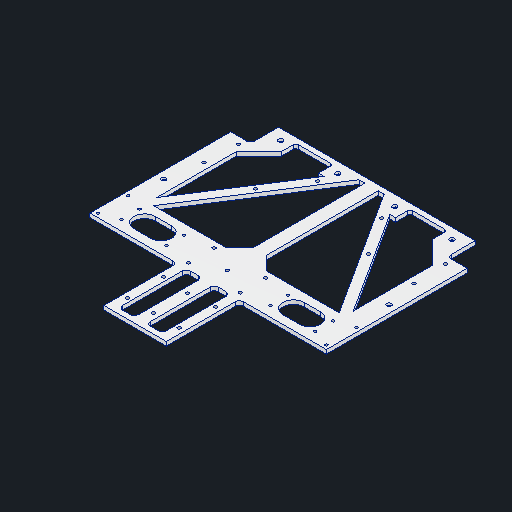
# Autodesk Inventor part: base
Saved by Autodesk Inventor 2023 (Build 270158000, 158)
## iProperties
Created: 2024-04-10
Part Number: base
Material: Aluminum 6061
Document SubType Name: Modeling
Designer: szymo
Density: 2.7 g/cm^3
Appearance: Aluminum - Flat
Mass: 95.625 g
Surface Area: 308.097 cm^2
Volume: 35.4167 cm^3
Author: szymo
Autodesk Inventor part; units mm, degrees
ref_plane "YZ Plane" through (0, 0, 0) normal (1, 0, 0) x (0, 1, 0)
ref_plane "XZ Plane" through (0, 0, 0) normal (0, 1, 0) x (-1, 0, 0)
ref_plane "XY Plane" through (0, 0, 0) normal (0, 0, 1) x (1, 0, 0)
sketch "Sketch2" plane through (0, 0, 0) normal (0, 1, 0) x (-1, 0, 0)
  line L0 (-89, 99) -> (89, 99)
  line L1 (89, 99) -> (89, -99)
  line L2 (89, -99) -> (-89, -99)
  line L3 (-89, -99) -> (-89, 99)
  line L4 (-89, 99) -> (89, -99) construction
  line L5 (89, 99) -> (-89, -99) construction
  line L6 (-89, 99) -> (89, 99)
  line L7 (89, 99) -> (89, -85)
  line L8 (89, -85) -> (-89, -85)
  line L9 (-89, -85) -> (-89, 99)
  line L10 (-4.5, 99) -> (-89, 99)
  line L11 (-89, 99) -> (-89, 42)
  line L12 (-89, 42) -> (-4.5, 42)
  line L13 (-4.5, 42) -> (-4.5, 99)
  line L14 (4.5, 99) -> (89, 99)
  line L15 (89, 99) -> (89, 42)
  line L16 (89, 42) -> (4.5, 42)
  line L17 (4.5, 42) -> (4.5, 99)
  line L18 (22.5, 77.5) -> (22.5, 66.5) projected
  line L19 (16.5, 66.5) -> (16.5, 77.5) projected
  line L20 (-22.5, 66.5) -> (-22.5, 77.5) projected
  line L21 (-16.5, 77.5) -> (-16.5, 66.5) projected
  line L22 (-23.5, 99) -> (-16.5, 99)
  line L23 (-16.5, 99) -> (-16.5, 42)
  line L24 (-16.5, 42) -> (-23.5, 42)
  line L25 (-23.5, 42) -> (-23.5, 99)
  line L26 (16.5, 99) -> (23.5, 99)
  line L27 (23.5, 99) -> (23.5, 42)
  line L28 (23.5, 42) -> (16.5, 42)
  line L29 (16.5, 42) -> (16.5, 99)
  line L30 (-89, 99) -> (89, 99)
  line L31 (89, 99) -> (89, 97)
  line L32 (89, 97) -> (-89, 97)
  line L33 (-89, 97) -> (-89, 99)
  line L34 (89, -85) -> (74, -85)
  line L35 (74, -85) -> (74, -64)
  line L36 (74, -64) -> (89, -64)
  line L37 (89, -64) -> (89, -85)
  line L38 (-89, -85) -> (-74, -85)
  line L39 (-74, -85) -> (-74, -64)
  line L40 (-74, -64) -> (-89, -64)
  line L41 (-89, -64) -> (-89, -85)
  line L42 (16.5, 97) -> (-16.5, 97)
  line L43 (-16.5, 97) -> (-16.5, 93)
  line L44 (-16.5, 93) -> (16.5, 93)
  line L45 (16.5, 93) -> (16.5, 97)
  line L46 (-84.4, -75) -> (-84.4, -71.5) projected
  line L47 (-84.4, -71.5) -> (-87, -71.5) projected
  line L48 (-87, -71.5) -> (-87, -75) projected
  line L49 (-87, -75) -> (-84.4, -75) projected
  line L50 (-79.6, -75) -> (-77, -75) projected
  line L51 (-77, -75) -> (-77, -71.5) projected
  line L52 (-77, -71.5) -> (-79.6, -71.5) projected
  line L53 (-79.6, -71.5) -> (-79.6, -75) projected
  line L54 (-75, -78) -> (-89, -78) projected
  line L55 (-89, -78) -> (-89, -63) projected
  line L56 (-89, -63) -> (-75, -63) projected
  line L57 (-75, -63) -> (-75, -78) projected
  circle A0 centre (-80.45, -67.25) radius 1.25 projected
  point P0 (0, 0)
  point P1 (4.5, 99)
  point P2 (-4.5, 99)
  point P3 (-89, 42)
  point P4 (89, 42)
  point P5 (4.5, 97)
  point P6 (-4.5, 97)
  point P7 (-16.5, 97)
  point P8 (-23.5, 97)
  point P9 (23.5, 97)
  point P10 (16.5, 98)
  point P11 (-4.5, 93)
  point P12 (4.5, 93)
  point P13 (16.5, 93)
  dimension "d8" = 178
  dimension "d9" = 198
  dimension "d10" = 14
  dimension "d11" = 84.5
  dimension "d13" = 84.5
  dimension "d17" = 9
  dimension "d18" = 2
  dimension "d19" = 15
  dimension "d20" = 21
  dimension "d21" = 15
  dimension "d22" = 21
  dimension "d75" = 55
  dimension "d76" = 55
  dimension "d77" = 7
  dimension "d78" = 7
  dimension "d79" = 4
  constraints: 84 end point, 20 parallel, 10 horizontal, 10 perpendicular, 10 point on line, 2 collinear, 2 midpoint, 5 other
  measures "d8" distance of L1.end L2.end
  measures "d9" distance of L0.end L1.end
  measures "d10" distance between parallel lines of L8 L2
  measures "d11" distance of L12.end L11.end
  measures "d13" distance of L15.end L16.end
  measures "d17" distance between parallel lines of L13 L17
  measures "d18" distance of L30.end L31.end
  measures "d19" distance of L35.end L36.end
  measures "d20" distance of L34.end L35.end
  measures "d21" distance of L40.end L39.end
  measures "d22" distance of L39.end L38.end
  measures "d75" distance between parallel lines of L32 L12
  measures "d76" distance between parallel lines of L32 L16
  measures "d77" distance between parallel lines of L23 L25
  measures "d78" distance between parallel lines of L27 L29
  measures "d79" distance of L43.end L42.end
extrude "Extrusion2" add sketch "Sketch2" along normal blind 3 contours L32 L23 L21 L12 L25 | L12 L13 L44 L17 L16 L1 L36 L35 L8 L39 L40 L57 L56 L3 | L32 L13 L44 L23 | L56 L57 L40 L3 | L32 L17 L44 L13 | L32 L29 L44 L17 | L32 L27 L16 L29 L19
fillet "Fillet5" radius 3 12 edges at (-16.5, 1.5, 42) (-4.5, 1.5, 42) (-23.5, 1.5, 42) (16.5, 1.5, 42) (-16.5, 1.5, 93) (-4.5, 1.5, 93) (4.5, 1.5, 93) (16.5, 1.5, 93) (4.5, 1.5, 42) (23.5, 1.5, 42) (74, 1.5, -64) (-74, 1.5, -64)
sketch "Sketch7" plane through (0, 3, 0) normal (0, 1, 0) x (1, 0, 0)
  circle A0 centre (78, 58.6725) radius 1.8 projected
  circle A1 centre (79, 33.8889) radius 1.8 projected
  circle A2 centre (42.4984, 36.1666) radius 1.8 projected
  circle A3 centre (24.1, 64.6) radius 1.6 projected
  circle A4 centre (24.1, 16.4) radius 1.6 projected
  circle A5 centre (-24.1, 16.4) radius 1.6 projected
  circle A6 centre (-24.1, 64.6) radius 1.6 projected
  circle A7 centre (-42.5, 36.1649) radius 1.8 projected
  circle A8 centre (-79, 33.8889) radius 1.8 projected
  circle A9 centre (-78, 58.6725) radius 1.8 projected
  circle A10 centre (19.5, -18.05) radius 1.8 projected
  circle A11 centre (19.5, -37.375) radius 1.8 projected
  circle A12 centre (19.5, -55.8) radius 1.8 projected
  circle A13 centre (19.4231, -83.3077) radius 1.8 projected
  circle A14 centre (0, -83.2) radius 1.8 projected
  circle A15 centre (-19.4231, -83.3077) radius 1.8 projected
  circle A16 centre (-19.5, -55.8) radius 1.8 projected
  circle A17 centre (0, -57.55) radius 1.8 projected
  circle A18 centre (0, -27.625) radius 1.8 projected
  circle A19 centre (-19.5, -37.375) radius 1.8 projected
  circle A20 centre (-19.5, -18.05) radius 1.8 projected
  point P0 (0, 0)
  point P1 (-19.5, -83.2)
  constraints: 20 coincident
hole "Hole3" at (19.4231, 3, 83.3077) at (0, 3, 83.2) at (-19.5, 3, 83.2) at (19.5, 3, 55.8) at (0, 3, 57.55) at (-19.5, 3, 55.8) at (-19.5, 3, 37.375) at (-19.5, 3, 18.05) at (0, 3, 27.625) at (19.5, 3, 37.375) at (19.5, 3, 18.05) at (79, 3, -33.8889) at (78, 3, -58.6725) at (42.4984, 3, -36.1666) at (24.1, 3, -16.4) at (-24.1, 3, -16.4) at (-24.1, 3, -64.6) at (24.1, 3, -64.6) at (-42.5, 3, -36.1649) at (-78, 3, -58.6725) at (-79, 3, -33.8889) direction (0, -1, 0) diameter 2.459 end through all thread size "M3x0.5" class "6H" standard "ISO Metric profile"
sketch "Sketch8" plane through (0, 3, 0) normal (0, 1, 0) x (1, 0, 0)
  circle A0 centre (72.95, -34.475) radius 1.45 projected
  circle A1 centre (72.95, -20.775) radius 1.45 projected
  circle A2 centre (39.125, -20.8375) radius 1.55 projected
  circle A3 centre (39.125, -34.4125) radius 1.55 projected
  circle A4 centre (-39.125, -20.8375) radius 1.55 projected
  circle A5 centre (-39.125, -34.4125) radius 1.55 projected
  circle A6 centre (-72.95, -34.475) radius 1.45 projected
  circle A7 centre (-72.95, -20.775) radius 1.45 projected
  circle A8 centre (86, -16.25) radius 2.3 projected
  circle A9 centre (86, -39) radius 2.3 projected
  circle A10 centre (86, 32.8889) radius 2.3 projected
  line L0 (89, -42) -> (83, -42) projected
  line L1 (89, 35.8889) -> (89, -42) projected
  line L2 (89, 35.8889) -> (83, 35.8889) projected
  line L3 (83, 29.8889) -> (83, 35.8889) projected
  line L4 (83, 29.8889) -> (87.4, 29.8889) projected
  line L5 (87.4, 29.8889) -> (87.4, 14.7889) projected
  line L6 (87.4, 14.7889) -> (79.4, 14.7889) projected
  line L7 (79.4, 2.7889) -> (79.4, 14.7889) projected
  line L8 (86, 2.7889) -> (79.4, 2.7889) projected
  line L9 (86, -13.25) -> (86, 2.7889) projected
  line L10 (86, -13.25) -> (83, -13.25) projected
  line L11 (83, -13.25) -> (83, -19.25) projected
  line L12 (83, -19.25) -> (86, -19.25) projected
  line L13 (86, -36) -> (86, -19.25) projected
  line L14 (86, -36) -> (83, -36) projected
  line L15 (83, -36) -> (83, -42) projected
  circle A11 centre (83.4, 10.7889) radius 2.6 projected
  circle A12 centre (-86, -39) radius 2.3 projected
  circle A13 centre (-86, -16.25) radius 2.3 projected
  line L16 (-86, -13.25) -> (-86, -0.1111) projected
  line L17 (-79.4, -0.1111) -> (-86, -0.1111) projected
  line L18 (-79.4, 11.8889) -> (-79.4, -0.1111) projected
  line L19 (-86, 11.8889) -> (-79.4, 11.8889) projected
  line L20 (-86, 11.8889) -> (-86, 29.8889) projected
  line L21 (-86, 29.8889) -> (-83, 29.8889) projected
  line L22 (-83, 29.8889) -> (-83, 35.8889) projected
  line L23 (-89, 35.8889) -> (-83, 35.8889) projected
  line L24 (-89, 35.8889) -> (-89, -42) projected
  line L25 (-89, -42) -> (-83, -42) projected
  line L26 (-83, -42) -> (-83, -36) projected
  line L27 (-83, -36) -> (-86, -36) projected
  line L28 (-86, -36) -> (-86, -19.25) projected
  line L29 (-86, -19.25) -> (-83, -19.25) projected
  line L30 (-83, -19.25) -> (-83, -13.25) projected
  line L31 (-83, -13.25) -> (-86, -13.25) projected
  circle A14 centre (-86, 32.8889) radius 2.3 projected
  circle A15 centre (-83.4, 7.8889) radius 2.6 projected
  line L32 (72.95, -34.475) -> (39.125, -12.8375)
  line L33 (72.95, -12.775) -> (39.125, -34.4125)
  line L34 (-39.125, -34.4125) -> (-72.95, -12.775)
  line L35 (-39.125, -12.8375) -> (-72.95, -34.4125)
  point P0 (0, 0)
  point P1 (56.0375, -23.5937)
  point P2 (-56.0375, -23.625)
  dimension "d90" = 8
  dimension "d91" = 8
  dimension "d92" = 8
  dimension "d93" = 8
  constraints: 12 coincident, 8 end point, 2 midpoint
  measures "d90" distance of A1.centre L33.start
  measures "d91" distance of L32.end A2.centre
  measures "d92" distance of point (-39.125, -20.837) L35.start
  measures "d93" distance of A7.centre L34.end
hole "Hole4" at (72.95, 3, 34.475) at (72.95, 3, 20.775) at (39.125, 3, 20.8375) at (39.125, 3, 34.4125) at (86, 3, 39) at (86, 3, 16.25) at (-86, 3, 39) at (-86, 3, 16.25) at (-72.95, 3, 20.775) at (-72.95, 3, 34.475) at (-39.125, 3, 34.4125) at (-39.125, 3, 20.8375) direction (0, -1, 0) diameter 2.013 end through all thread size "M2.5x0.45" class "6H" standard "ISO Metric profile"
sketch "Sketch9" plane through (0, 0, 0) normal (0, -1, 0) x (1, 0, 0)
  circle A0 centre (64.5, -77) radius 1.2295 projected
  circle A1 centre (21.5, -77) radius 1.2295 projected
  circle A2 centre (-21.5, -77) radius 1.2295 projected
  circle A3 centre (-64.5, -77) radius 1.2295 projected
  circle A4 centre (-83.4, -7.8889) radius 2.6 projected
  circle A5 centre (83.4, -10.7889) radius 2.6 projected
  point P0 (0, 0)
  constraints: 6 coincident
hole "Hole5" at (-83.4, 0, -7.8889) at (83.4, 0, -10.7889) at (64.5, 0, -77) at (21.5, 0, -77) at (-21.5, 0, -77) at (-64.5, 0, -77) direction (0, 1, 0) diameter 3.6 end through all countersink diameter 6.6 countersink angle 90 clearance for "Countersunk Flat Head Screw ISO 2009/7046" size "M3" standard "ISO"
sketch "Sketch11" plane through (0, 0, 0) normal (0, -1, 0) x (1, 0, 0)
  circle A0 centre (-21.5, -77) radius 3.3
  circle A1 centre (64.5, -77) radius 3.3
  circle A2 centre (-83.4, -7.8889) radius 3.3
  circle A3 centre (83.4, -10.7889) radius 3.3
  circle A4 centre (21.5, -77) radius 3.3
  circle A5 centre (-64.5, -77) radius 3.3
  circle A6 centre (-39.125, 34.4125) radius 1.0065
  circle A7 centre (-72.95, 20.775) radius 1.0065
  circle A8 centre (-86, 39) radius 1.0065
  circle A9 centre (86, 39) radius 1.0065
  circle A10 centre (39.125, 20.8375) radius 1.0065
  circle A11 centre (72.95, 34.475) radius 1.0065
  circle A12 centre (72.95, 20.775) radius 1.0065
  circle A13 centre (39.125, 34.4125) radius 1.0065
  circle A14 centre (86, 16.25) radius 1.0065
  circle A15 centre (-86, 16.25) radius 1.0065
  circle A16 centre (-72.95, 34.475) radius 1.0065
  circle A17 centre (-39.125, 20.8375) radius 1.0065
  circle A18 centre (-78, -58.6725) radius 1.2295
  circle A19 centre (24.1, -64.6) radius 1.2295
  circle A20 centre (-24.1, -16.4) radius 1.2295
  circle A21 centre (42.4984, -36.1666) radius 1.2295
  circle A22 centre (79, -33.8889) radius 1.2295
  circle A23 centre (19.5, 37.375) radius 1.2295
  circle A24 centre (-19.5, 18.05) radius 1.2295
  circle A25 centre (-19.5, 55.8) radius 1.2295
  circle A26 centre (19.5, 55.8) radius 1.2295
  circle A27 centre (0, 83.2) radius 1.2295
  circle A28 centre (19.4231, 83.3077) radius 1.2295
  circle A29 centre (-19.5, 83.2) radius 1.2295
  circle A30 centre (0, 57.55) radius 1.2295
  circle A31 centre (-19.5, 37.375) radius 1.2295
  circle A32 centre (0, 27.625) radius 1.2295
  circle A33 centre (19.5, 18.05) radius 1.2295
  circle A34 centre (78, -58.6725) radius 1.2295
  circle A35 centre (24.1, -16.4) radius 1.2295
  circle A36 centre (-24.1, -64.6) radius 1.2295
  circle A37 centre (-42.5, -36.1649) radius 1.2295
  circle A38 centre (-79, -33.8889) radius 1.2295
  arc A39 (-13.5, 93) -> (-16.5, 90) centre (-13.5, 90) ccw
  line L0 (-7.5, 93) -> (-13.5, 93)
  arc A40 (-4.5, 90) -> (-7.5, 93) centre (-7.5, 90) ccw
  line L1 (-4.5, 45) -> (-4.5, 90)
  arc A41 (-7.5, 42) -> (-4.5, 45) centre (-7.5, 45) ccw
  line L2 (-13.5, 42) -> (-7.5, 42)
  arc A42 (-16.5, 45) -> (-13.5, 42) centre (-13.5, 45) ccw
  line L3 (-16.5, 90) -> (-16.5, 45)
  arc A43 (16.5, 90) -> (13.5, 93) centre (13.5, 90) ccw
  line L4 (16.5, 45) -> (16.5, 90)
  arc A44 (13.5, 42) -> (16.5, 45) centre (13.5, 45) ccw
  line L5 (7.5, 42) -> (13.5, 42)
  arc A45 (4.5, 45) -> (7.5, 42) centre (7.5, 45) ccw
  line L6 (4.5, 90) -> (4.5, 45)
  arc A46 (7.5, 93) -> (4.5, 90) centre (7.5, 90) ccw
  line L7 (13.5, 93) -> (7.5, 93)
  line L8 (-23.5, 97) -> (23.5, 97)
  line L9 (-23.5, 45) -> (-23.5, 97)
  arc A47 (-26.5, 42) -> (-23.5, 45) centre (-26.5, 45) ccw
  line L10 (-89, 42) -> (-26.5, 42)
  line L11 (-89, -64) -> (-89, 42)
  line L12 (-77, -64) -> (-89, -64)
  arc A48 (-74, -67) -> (-77, -64) centre (-77, -67) ccw
  line L13 (-74, -85) -> (-74, -67)
  line L14 (74, -85) -> (-74, -85)
  line L15 (74, -67) -> (74, -85)
  arc A49 (77, -64) -> (74, -67) centre (77, -67) ccw
  line L16 (89, -64) -> (77, -64)
  line L17 (89, 42) -> (89, -64)
  line L18 (26.5, 42) -> (89, 42)
  arc A50 (23.5, 45) -> (26.5, 42) centre (26.5, 45) ccw
  line L19 (23.5, 97) -> (23.5, 45)
  circle A51 centre (-42.5, -36.1649) radius 1.8
  line L20 (-86, 0.1111) -> (-86, 42)
  line L21 (-89, 42) -> (-86, 42)
  line L22 (-89, 42) -> (-89, 38.75)
  line L23 (-89, 38.75) -> (-89, 13.5)
  line L24 (-89, 13.5) -> (-89, -81)
  line L25 (-89, -81) -> (-83, -81)
  line L26 (-83, -81) -> (-83, -75)
  line L27 (-83, -75) -> (-73, -75)
  line L28 (-73, -75) -> (-73, -53.3451)
  line L29 (-73, -53.3451) -> (-67, -53.3451)
  line L30 (-67, -53.3451) -> (-67, -42.9318)
  line L31 (-76.801, -42.9318) -> (-67, -42.9318)
  line L32 (-75, -34.8889) -> (-75, -29.8889)
  line L33 (-86, -29.8889) -> (-75, -29.8889)
  line L34 (-86, -29.8889) -> (-86, -11.8889)
  line L35 (-79.4, -11.8889) -> (-86, -11.8889)
  line L36 (-79.4, 0.1111) -> (-79.4, -11.8889)
  line L37 (-86, 0.1111) -> (-79.4, 0.1111)
  circle A52 centre (-83.5, -70.5) radius 1.75
  circle A53 centre (-79, -33.8889) radius 1.8
  circle A54 centre (-83.4, -7.8889) radius 2.6
  circle A55 centre (-78, -58.6725) radius 1.8
  circle A56 centre (78, -58.6725) radius 1.8
  circle A57 centre (79, -33.8889) radius 1.8
  circle A58 centre (83.4, -10.7889) radius 2.6
  circle A59 centre (80.5, -70.5) radius 1.75
  circle A60 centre (42.4984, -36.1666) radius 1.8
  spline S0 degree 2 poles (89, 38.051) (88.5208, 39.25) (89, 40.449) knots 0 0 0 1 1 1 weights 1 1.090909 1
  line L38 (89, 42) -> (89, 40.449)
  line L39 (89, 42) -> (86, 42)
  line L40 (86, -2.7889) -> (86, 42)
  line L41 (79.4, -2.7889) -> (86, -2.7889)
  line L42 (79.4, -14.7889) -> (79.4, -2.7889)
  line L43 (86, -14.7889) -> (79.4, -14.7889)
  line L44 (86, -16.7889) -> (86, -14.7889)
  line L45 (86, -27.8889) -> (86, -16.7889)
  line L46 (86, -29.8889) -> (86, -27.8889)
  ellipse E0 centre (76.799, -27.2986) end of major axis (76.7969, -11.6653) minor radius 1.851 (76.801, -42.9318) -> (77.5308, -41.6649) ccw
  line L47 (76.801, -42.9318) -> (67, -42.9318)
  line L48 (67, -53.3451) -> (67, -42.9318)
  line L49 (73, -53.3451) -> (67, -53.3451)
  line L50 (73, -75) -> (73, -53.3451)
  line L51 (83, -75) -> (73, -75)
  line L52 (83, -81) -> (83, -75)
  line L53 (89, -81) -> (83, -81)
  line L54 (89, 14.801) -> (89, -81)
  spline S1 degree 2 poles (89, 14.801) (88.5208, 16) (89, 17.199) knots 0 0 0 1 1 1 weights 1 1.090909 1
  line L55 (89, 38.051) -> (89, 17.199)
  line L56 (27.5, -68) -> (27.5, -13)
  line L57 (27.5, -13) -> (-27.5, -13)
  line L58 (-27.5, -13) -> (-27.5, -68)
  line L59 (-27.5, -68) -> (27.5, -68)
  circle A61 centre (24.1, -64.6) radius 1.6
  circle A62 centre (24.1, -16.4) radius 1.6
  circle A63 centre (-24.1, -64.6) radius 1.6
  circle A64 centre (-24.1, -16.4) radius 1.6
  circle A65 centre (21.5, -77) radius 1.2295
  circle A66 centre (-64.5, -77) radius 1.2295
  circle A67 centre (-21.5, -77) radius 1.2295
  circle A68 centre (64.5, -77) radius 1.2295
  line L60 (-72, -70) -> (-72, -79)
  arc A69 (-74, -81) -> (-72, -79) centre (-74, -79) ccw
  line L61 (-74, -81) -> (-89, -81)
  line L62 (-89, -81) -> (-89, -85)
  line L63 (-89, -85) -> (89, -85)
  line L64 (89, -81) -> (89, -85)
  line L65 (89, -81) -> (74, -81)
  arc A70 (72, -79) -> (74, -81) centre (74, -79) ccw
  line L66 (72, -79) -> (72, -70)
  line L67 (57, -70) -> (72, -70)
  line L68 (57, -70) -> (57, -79)
  arc A71 (55, -81) -> (57, -79) centre (55, -79) ccw
  line L69 (55, -81) -> (31, -81)
  arc A72 (29, -79) -> (31, -81) centre (31, -79) ccw
  line L70 (29, -79) -> (29, -70)
  line L71 (14, -70) -> (29, -70)
  line L72 (14, -70) -> (14, -79)
  arc A73 (12, -81) -> (14, -79) centre (12, -79) ccw
  line L73 (12, -81) -> (-12, -81)
  arc A74 (-14, -79) -> (-12, -81) centre (-12, -79) ccw
  line L74 (-14, -79) -> (-14, -70)
  line L75 (-29, -70) -> (-14, -70)
  line L76 (-29, -70) -> (-29, -79)
  arc A75 (-31, -81) -> (-29, -79) centre (-31, -79) ccw
  line L77 (-31, -81) -> (-55, -81)
  arc A76 (-57, -79) -> (-55, -81) centre (-55, -79) ccw
  line L78 (-57, -79) -> (-57, -70)
  line L79 (-72, -70) -> (-57, -70)
  line L80 (-89, -85) -> (-89, -99)
  line L81 (-89, -99) -> (89, -99)
  line L82 (89, -85) -> (89, -99)
  line L83 (-89, -85) -> (89, -85)
  circle A77 centre (72.95, 34.475) radius 1.45
  circle A78 centre (72.95, 20.775) radius 1.45
  circle A79 centre (39.125, 34.4125) radius 1.55
  circle A80 centre (39.125, 20.8375) radius 1.55
  spline S2 degree 3 poles (65.7, 23.025) (65.7, 22.8819) (65.6837, 22.6312) (65.6334, 22.3458) (65.5819, 22.1333) (65.5405, 21.9923) (65.48, 21.8179) (65.4239, 21.6792) (65.3456, 21.5106) (65.2769, 21.3802) (65.184, 21.2227) (65.1043, 21.1011) (64.9982, 20.9549) (64.9083, 20.8425) (64.7662, 20.6811) (64.615, 20.5299) (64.3941, 20.3423) (64.2146, 20.2128) (64.0241, 20.0935) (63.8917, 20.0193) (63.7367, 19.9424) (63.63, 19.8951) (63.5206, 19.8513) (63.4473, 19.8241) (63.3368, 19.7865) (63.2255, 19.7528) (63.02, 19.6999) (62.7939, 19.6576) (62.4526, 19.6224) (62.1474, 19.6224) (61.8061, 19.6576) (61.58, 19.6999) (61.3745, 19.7528) (61.2632, 19.7865) (61.1527, 19.8241) (61.0794, 19.8513) (60.97, 19.8951) (60.8633, 19.9424) (60.7083, 20.0193) (60.5759, 20.0935) (60.3854, 20.2128) (60.2059, 20.3423) (59.985, 20.5299) (59.8338, 20.6811) (59.6917, 20.8425) (59.6018, 20.9549) (59.4957, 21.1011) (59.416, 21.2227) (59.3231, 21.3802) (59.2544, 21.5106) (59.1761, 21.6792) (59.12, 21.8179) (59.0595, 21.9923) (59.0181, 22.1333) (58.9666, 22.3458) (58.9163, 22.6312) (58.9, 22.8819) (58.9, 23.025) knots 0.368505 0.368505 0.368505 0.368505 0.400174 0.423925 0.431842 0.447677 0.455594 0.471428 0.479345 0.49518 0.503097 0.518931 0.526849 0.542683 0.5506 0.574352 0.590186 0.613938 0.621855 0.637689 0.645607 0.657482 0.661441 0.669358 0.673317 0.685193 0.69311 0.716861 0.732696 0.764365 0.780199 0.803951 0.811868 0.823744 0.827702 0.835619 0.839578 0.851454 0.859371 0.875205 0.883123 0.906874 0.922709 0.94646 0.954377 0.970212 0.978129 0.993963 1.00188 1.017715 1.025632 1.041466 1.049384 1.065218 1.073135 1.096887 1.128556 1.128556 1.128556 1.128556
  line L84 (58.9, 23.025) -> (58.9, 32.225)
  spline S3 degree 3 poles (58.9, 32.225) (58.9, 32.3681) (58.9163, 32.6188) (58.9666, 32.9042) (59.0181, 33.1167) (59.0595, 33.2577) (59.12, 33.4321) (59.1761, 33.5708) (59.2544, 33.7394) (59.3231, 33.8698) (59.416, 34.0273) (59.4957, 34.1489) (59.6018, 34.2951) (59.6917, 34.4075) (59.8338, 34.5689) (59.985, 34.7201) (60.2059, 34.9077) (60.3854, 35.0372) (60.5759, 35.1565) (60.7083, 35.2307) (60.8633, 35.3076) (60.97, 35.3549) (61.0794, 35.3987) (61.1527, 35.4259) (61.2632, 35.4635) (61.3745, 35.4972) (61.58, 35.5501) (61.8061, 35.5924) (62.1474, 35.6276) (62.4526, 35.6276) (62.7939, 35.5924) (63.02, 35.5501) (63.2255, 35.4972) (63.3368, 35.4635) (63.4473, 35.4259) (63.5206, 35.3987) (63.63, 35.3549) (63.7367, 35.3076) (63.8917, 35.2307) (64.0241, 35.1565) (64.2146, 35.0372) (64.3941, 34.9077) (64.615, 34.7201) (64.7662, 34.5689) (64.9083, 34.4075) (64.9982, 34.2951) (65.1043, 34.1489) (65.184, 34.0273) (65.2769, 33.8698) (65.3456, 33.7394) (65.4239, 33.5708) (65.48, 33.4321) (65.5405, 33.2577) (65.5819, 33.1167) (65.6334, 32.9042) (65.6837, 32.6188) (65.7, 32.3681) (65.7, 32.225) knots -0.380025 -0.380025 -0.380025 -0.380025 -0.348357 -0.324605 -0.316688 -0.300853 -0.292936 -0.277102 -0.269185 -0.25335 -0.245433 -0.229599 -0.221682 -0.205847 -0.19793 -0.174178 -0.158344 -0.134592 -0.126675 -0.110841 -0.102924 -0.091048 -0.087089 -0.079172 -0.075213 -0.063338 -0.05542 -0.031669 -0.015834 0.015834 0.031669 0.05542 0.063338 0.075213 0.079172 0.087089 0.091048 0.102924 0.110841 0.126675 0.134592 0.158344 0.174178 0.19793 0.205847 0.221682 0.229599 0.245433 0.25335 0.269185 0.277102 0.292936 0.300853 0.316688 0.324605 0.348357 0.380025 0.380025 0.380025 0.380025
  line L85 (65.7, 32.225) -> (65.7, 23.025)
  line L86 (27.2, 42) -> (86, 42)
  line L87 (27.2, 13.25) -> (27.2, 42)
  line L88 (27.2, 13.25) -> (86, 13.25)
  line L89 (86, 42) -> (86, 13.25)
  circle A81 centre (-72.95, 34.475) radius 1.45
  circle A82 centre (-72.95, 20.775) radius 1.45
  circle A83 centre (-39.125, 34.4125) radius 1.55
  circle A84 centre (-39.125, 20.8375) radius 1.55
  spline S4 degree 3 poles (-65.7, 23.025) (-65.7, 22.8819) (-65.6837, 22.6312) (-65.6334, 22.3458) (-65.5819, 22.1333) (-65.5405, 21.9923) (-65.48, 21.8179) (-65.4239, 21.6792) (-65.3456, 21.5106) (-65.2769, 21.3802) (-65.184, 21.2227) (-65.1043, 21.1011) (-64.9982, 20.9549) (-64.9083, 20.8425) (-64.7662, 20.6811) (-64.615, 20.5299) (-64.3941, 20.3423) (-64.2146, 20.2128) (-64.0241, 20.0935) (-63.8917, 20.0193) (-63.7367, 19.9424) (-63.63, 19.8951) (-63.5206, 19.8513) (-63.4473, 19.8241) (-63.3368, 19.7865) (-63.2255, 19.7528) (-63.02, 19.6999) (-62.7939, 19.6576) (-62.4526, 19.6224) (-62.1474, 19.6224) (-61.8061, 19.6576) (-61.58, 19.6999) (-61.3745, 19.7528) (-61.2632, 19.7865) (-61.1527, 19.8241) (-61.0794, 19.8513) (-60.97, 19.8951) (-60.8633, 19.9424) (-60.7083, 20.0193) (-60.5759, 20.0935) (-60.3854, 20.2128) (-60.2059, 20.3423) (-59.985, 20.5299) (-59.8338, 20.6811) (-59.6917, 20.8425) (-59.6018, 20.9549) (-59.4957, 21.1011) (-59.416, 21.2227) (-59.3231, 21.3802) (-59.2544, 21.5106) (-59.1761, 21.6792) (-59.12, 21.8179) (-59.0595, 21.9923) (-59.0181, 22.1333) (-58.9666, 22.3458) (-58.9163, 22.6312) (-58.9, 22.8819) (-58.9, 23.025) knots 0.368505 0.368505 0.368505 0.368505 0.400174 0.423925 0.431842 0.447677 0.455594 0.471428 0.479345 0.49518 0.503097 0.518931 0.526849 0.542683 0.5506 0.574352 0.590186 0.613938 0.621855 0.637689 0.645607 0.657482 0.661441 0.669358 0.673317 0.685193 0.69311 0.716861 0.732696 0.764365 0.780199 0.803951 0.811868 0.823744 0.827702 0.835619 0.839578 0.851454 0.859371 0.875205 0.883123 0.906874 0.922709 0.94646 0.954377 0.970212 0.978129 0.993963 1.00188 1.017715 1.025632 1.041466 1.049384 1.065218 1.073135 1.096887 1.128556 1.128556 1.128556 1.128556
  line L90 (-65.7, 32.225) -> (-65.7, 23.025)
  spline S5 degree 3 poles (-58.9, 32.225) (-58.9, 32.3681) (-58.9163, 32.6188) (-58.9666, 32.9042) (-59.0181, 33.1167) (-59.0595, 33.2577) (-59.12, 33.4321) (-59.1761, 33.5708) (-59.2544, 33.7394) (-59.3231, 33.8698) (-59.416, 34.0273) (-59.4957, 34.1489) (-59.6018, 34.2951) (-59.6917, 34.4075) (-59.8338, 34.5689) (-59.985, 34.7201) (-60.2059, 34.9077) (-60.3854, 35.0372) (-60.5759, 35.1565) (-60.7083, 35.2307) (-60.8633, 35.3076) (-60.97, 35.3549) (-61.0794, 35.3987) (-61.1527, 35.4259) (-61.2632, 35.4635) (-61.3745, 35.4972) (-61.58, 35.5501) (-61.8061, 35.5924) (-62.1474, 35.6276) (-62.4526, 35.6276) (-62.7939, 35.5924) (-63.02, 35.5501) (-63.2255, 35.4972) (-63.3368, 35.4635) (-63.4473, 35.4259) (-63.5206, 35.3987) (-63.63, 35.3549) (-63.7367, 35.3076) (-63.8917, 35.2307) (-64.0241, 35.1565) (-64.2146, 35.0372) (-64.3941, 34.9077) (-64.615, 34.7201) (-64.7662, 34.5689) (-64.9083, 34.4075) (-64.9982, 34.2951) (-65.1043, 34.1489) (-65.184, 34.0273) (-65.2769, 33.8698) (-65.3456, 33.7394) (-65.4239, 33.5708) (-65.48, 33.4321) (-65.5405, 33.2577) (-65.5819, 33.1167) (-65.6334, 32.9042) (-65.6837, 32.6188) (-65.7, 32.3681) (-65.7, 32.225) knots -0.380025 -0.380025 -0.380025 -0.380025 -0.348357 -0.324605 -0.316688 -0.300853 -0.292936 -0.277102 -0.269185 -0.25335 -0.245433 -0.229599 -0.221682 -0.205847 -0.19793 -0.174178 -0.158344 -0.134592 -0.126675 -0.110841 -0.102924 -0.091048 -0.087089 -0.079172 -0.075213 -0.063338 -0.05542 -0.031669 -0.015834 0.015834 0.031669 0.05542 0.063338 0.075213 0.079172 0.087089 0.091048 0.102924 0.110841 0.126675 0.134592 0.158344 0.174178 0.19793 0.205847 0.221682 0.229599 0.245433 0.25335 0.269185 0.277102 0.292936 0.300853 0.316688 0.324605 0.348357 0.380025 0.380025 0.380025 0.380025
  line L91 (-58.9, 23.025) -> (-58.9, 32.225)
  line L92 (-27.2, 42) -> (-86, 42)
  line L93 (-86, 42) -> (-86, 13.25)
  line L94 (-27.2, 13.25) -> (-86, 13.25)
  line L95 (-27.2, 13.25) -> (-27.2, 42)
  line L96 (-22.5, 14.25) -> (22.5, 14.25)
  line L97 (22.5, 14.25) -> (22.5, 13.25)
  line L98 (-22.5, 13.25) -> (22.5, 13.25)
  line L99 (-22.5, 14.25) -> (-22.5, 13.25)
  line L100 (-27.2, 13.25) -> (-27.2, 42)
  line L101 (-27.2, 13.25) -> (-22.7, 13.25)
  line L102 (-22.7, 13.25) -> (-22.7, 42)
  line L103 (-27.2, 42) -> (-22.7, 42)
  line L104 (27.2, 13.25) -> (27.2, 42)
  line L105 (27.2, 42) -> (22.7, 42)
  line L106 (22.7, 13.25) -> (22.7, 42)
  line L107 (27.2, 13.25) -> (22.7, 13.25)
  line L108 (-77.0142, -3.75) -> (-9.0142, -3.75)
  line L109 (-9.0142, -3.75) -> (-9.0142, 11.25)
  line L110 (-9.0142, 11.25) -> (-77.0142, 11.25)
  line L111 (-77.0142, 11.25) -> (-77.0142, -3.75)
  line L112 (77.6433, -8.75) -> (11.6433, -8.75)
  line L113 (77.6433, 11.25) -> (77.6433, -8.75)
  line L114 (11.6433, 11.25) -> (77.6433, 11.25)
  line L115 (11.6433, -8.75) -> (11.6433, 11.25)
  line L116 (-74, -85) -> (74, -85)
  line L117 (74, -85) -> (74, -70)
  line L118 (-74, -70) -> (-74, -85)
  line L119 (-89, -64) -> (-74, -64)
  line L120 (-74, -64) -> (-74, 42)
  line L121 (-74, 42) -> (-89, 42)
  line L122 (-89, 42) -> (-89, -64)
  line L123 (89, 42) -> (89, -64)
  line L124 (89, -64) -> (74, -64)
  line L125 (74, -64) -> (74, 42)
  line L126 (74, 42) -> (89, 42)
  line L127 (89, 42) -> (89, -64)
  line L128 (-74, 13.25) -> (74, 13.25)
  line L129 (0, -102.1989) -> (-74, 13.25) construction
  line L130 (0, -102.1989) -> (74, 13.25) construction
  line L131 (-15.1814, -85) -> (-74, 6.7642)
  line L132 (15.1814, -85) -> (74, 6.7642)
  line L133 (0, -95.7131) -> (69.8427, 13.25)
  line L134 (0, -95.7131) -> (-69.8427, 13.25)
  line L135 (0, 13.25) -> (0, -95.7131) construction
  line L136 (5, -87.9125) -> (5, 3.25)
  line L137 (-5, 3.25) -> (-5, -87.9125)
  line L138 (-5, 3.25) -> (-15, 13.25)
  line L139 (5, 3.25) -> (15, 13.25)
  circle A85 centre (-42.5, -36.1649) radius 1.2295
  line L140 (-86, 27.625) -> (-22.7, 27.625)
  circle A86 centre (-62.3, 27.625) radius 8
  circle A87 centre (-49.775, 27.625) radius 8
  line L141 (-62.3, 35.625) -> (-49.775, 35.625)
  line L142 (-49.775, 19.625) -> (-62.3, 19.625)
  line L143 (0, 57.55) -> (0, 27.625) construction
  line L144 (27.2, 27.625) -> (86, 27.625)
  circle A88 centre (62.3, 27.625) radius 8
  circle A89 centre (49.775, 27.625) radius 8
  line L145 (62.3, 35.625) -> (49.775, 35.625)
  line L146 (49.775, 19.625) -> (62.3, 19.625)
  line L147 (-57, -70) -> (-74, -53)
  line L148 (57, -70) -> (74, -53)
  point P0 (-9.0142, 8.7685)
  point P1 (11.6433, 8.7685)
  point P2 (11.6433, 9.8933)
  point P3 (74, -42.9318)
  point P4 (-74, -42.9318)
  point P5 (27.5, -65.7814)
  point P6 (-27.5, -65.7814)
  point P7 (-69.8427, 13.25)
  point P8 (-86, 17.2565)
  point P9 (-86, 15.2435)
  point P10 (-86, 40.0065)
  point P11 (-86, 37.9935)
  point P12 (-74, 33.475)
  point P13 (-74, 35.475)
  point P14 (-74, 19.775)
  point P15 (-74, 21.775)
  point P16 (86, 37.9935)
  point P17 (86, 40.0065)
  point P18 (86, 15.2435)
  point P19 (86, 17.2565)
  point P20 (74, 21.775)
  point P21 (74, 19.775)
  point P22 (74, 35.475)
  point P23 (74, 33.475)
  point P24 (26.078, -68)
  point P25 (-26.078, -68)
  point P26 (-27.5, -52.8097)
  point P27 (-17.7634, -68)
  point P28 (17.7634, -68)
  point P29 (27.5, -52.8097)
  point P30 (5, -13)
  point P31 (-5, -13)
  point P32 (-24.796, -70)
  point P33 (24.796, -70)
  point P34 (-5, -68)
  point P35 (5, -68)
  point P36 (5, -81)
  point P37 (9.4307, -81)
  point P38 (-5, -81)
  point P39 (-9.4307, -81)
  dimension "d146" = 15
  dimension "d147" = 15
  dimension "d151" = 3.5
  dimension "d152" = 7
  dimension "d153" = 7
  dimension "d154" = 3.5
  dimension "d167" = 5
  dimension "d169" = 10
  dimension "d170" = 45
  dimension "d171" = 45
  dimension "d183" = 14.375
  dimension "d184" = 14.375
  dimension "d185" = 3.4
  dimension "d186" = 3.4
  dimension "d188" = 10.65
  dimension "d189" = 10.65
  dimension "d190" = 3.4
  dimension "d191" = 3.4
  dimension "d192" = 10.65
  dimension "d193" = 10.65
  dimension "d204" = 10
  dimension "d205" = 10
  dimension "d206" = 45
  dimension "d207" = 45
  constraints: 64 end point, 22 point on line, 11 parallel, 8 point on circle, 5 midpoint, 5 perpendicular, 4 centre point, 4 tangent, 3 horizontal, 2 equal radius, 2 vertical, 1 collinear, 7 other
  measures "d146" distance of L121.end L120.end
  measures "d147" distance of L125.end L126.end
  measures "d151" distance between parallel lines of L129 L131
  measures "d152" distance between parallel lines of L131 L134
  measures "d153" distance between parallel lines of L133 L132
  measures "d154" distance between parallel lines of L130 L132
  measures "d167" distance between parallel lines of L135 L136
  measures "d169" distance between parallel lines of L137 L136
  measures "d170" angle of L128 L138
  measures "d171" angle of L128 L139
  measures "d183" distance between parallel lines of L92 L140
  measures "d184" distance between parallel lines of L140 L94
  measures "d185" distance from line of A86.centre L91
  measures "d186" distance from line of L90 A86.centre
  measures "d188" horizontal distance of A7.centre A86.centre
  measures "d189" horizontal distance of A87.centre A17.centre
  measures "d190" distance from line of L85 A88.centre
  measures "d191" distance from line of L84 A88.centre
  measures "d192" horizontal distance of A88.centre A12.centre
  measures "d193" horizontal distance of A10.centre A89.centre
  measures "d204" distance from line of L128 L137.start
  measures "d205" distance from line of L128 L136.end
  measures "d206" angle of L148 L67
  measures "d207" angle of L147 L79
extrude "Extrusion5" cut sketch "Sketch11" against normal up to next contours L75 L76 A75 L77 A76 L78 L147 L28 L29 L30 L31 L120 L108 L131 L58 L59 | L134 L59 L137 L73 L74 L75 | L75 L74 L134 | L59 L58 L131 | L134 L58 L57 L137 L59 | L134 L108 L109 L138 L137 L57 L58 | L108 L120 L131 | L136 L57 L56 L133 L59 | L59 L133 L71 L72 L73 L136 | L134 L110 L138 L109 L108 | L136 L139 L115 L112 L133 L56 L57 | L134 L94 L101 L128 L98 L138 L110 | L31 L30 L29 L28 L147 L120 | L132 L56 L59 | L59 L56 L132 L112 L125 L47 L48 L49 L50 L148 L68 A71 L69 A72 L70 L71 | L133 L72 L71 | L112 L115 L139 L114 L133 | L132 L125 L112 | L114 L139 L98 L128 L107 L88 L133 | L20 A15 | A87 A86 L140 | L140 A86 A87 | A8 L20 | L125 L148 L50 L49 L48 L47 | A86 A87 L140 | L140 A87 A86 | A87 A86 L141 | L142 A86 A87 | A86 S5 L90 L140 | L140 L90 S4 A86 | A87 A86 S4 L91 L140 | L140 L91 S5 A86 A87 | S5 L91 L140 L90 | S4 L90 L140 L91 | A89 A88 L144 | L144 A88 A89 | A88 A89 L144 | L144 A89 A88 | L145 A88 A89 | A89 A88 L146 | A88 S2 L85 L144 | L144 L85 S3 A88 | A89 A88 S3 L84 L144 | L144 L84 S2 A88 A89 | S3 L85 L144 L84 | S2 L84 L144 L85 | A19 | A20 | A35 | A36 | A62 | A64 picked at (-85.6977, 16.3956) picked at (-85.6977, 39.1456)
equation "\"d11\" = d13"
body "Solid2"
